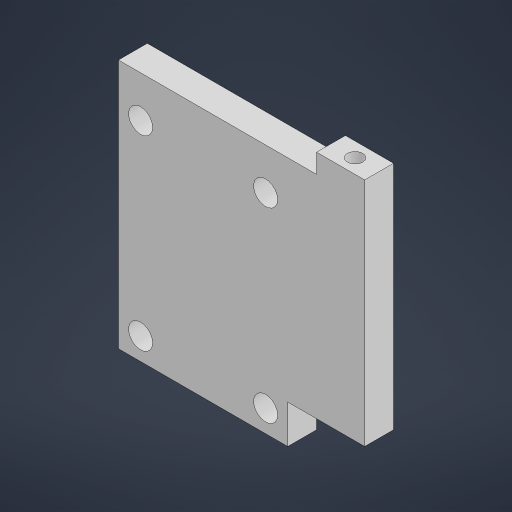
# Autodesk Inventor part: KickerMount_R
Saved by Autodesk Inventor 2024.2 (Build 282272000, 272)
## iProperties
Created: 2023-12-22
Part Number: KickerMount_R
Material: 一般
Document SubType Name: Modeling
Designer: Hanaoka
Density: 1 g/cm^3
Appearance: 既定
Author: Hanaoka
Autodesk Inventor part; units mm, degrees
ref_plane "YZ Plane" through (0, 0, 0) normal (1, 0, 0) x (0, 1, 0)
ref_plane "XZ Plane" through (0, 0, 0) normal (0, 1, 0) x (-1, 0, 0)
ref_plane "作業平面1" through (0, 0, 0) normal (0, 0, 1) x (1, 0, 0)
sketch "スケッチ1" plane through (0, 0, 0) normal (0, 0, 1) x (1, 0, 0)
  circle A0 centre (-6, -21.7) radius 1.25 projected
  circle A1 centre (-19, -21.7) radius 1.25 projected
  circle A2 centre (-19, -2.3) radius 1.25 projected
  circle A3 centre (-6, -2.3) radius 1.25 projected
  line L0 (0, -24) -> (-27.3, -24) projected
  line L1 (-3.7, -24) -> (-3.7, 2)
  line L2 (-3.7, 2) -> (-21.3, 2)
  line L3 (-21.3, 2) -> (-21.3, -24)
  circle A4 centre (-6, -21.7) radius 2.3 construction
  circle A5 centre (-19, -21.7) radius 2.3 construction
  line L4 (-3.7, -20) -> (4.3, -20)
  line L5 (4.3, -20) -> (4.3, 4)
  line L6 (4.3, 4) -> (-0.7, 4)
  line L7 (-0.7, 4) -> (-0.7, 2)
  line L8 (-0.7, 2) -> (-3.7, 2)
  point P0 (0, 0)
  dimension "d0" = 26
  dimension "d3" = 3
  dimension "d4" = 5
  dimension "d5" = 2
  dimension "d6" = 24
  constraints: 16 end point, 3 perpendicular, 3 point on line, 3 tangent, 2 centre point, 2 coincident, 2 horizontal, 2 vertical, 1 collinear, 1 equal radius
  measures "d0" distance of L1.start L1.end
  measures "d3" distance of L7.end L1.end
  measures "d4" distance of L5.end L6.end
  measures "d5" distance of L6.end L7.end
  measures "d6" distance of L4.end L5.end
extrude "押し出し1" add sketch "スケッチ1" along normal blind 3
sketch "スケッチ2" plane through (-0.7, 4, 0) normal (0, 1, 0) x (1, 0, 0)
  line L0 (5, 0) -> (0, 0) projected
  line L1 (0, 0) -> (0, -3) projected
  line L2 (5, -3) -> (0, -3) projected
  line L3 (5, 0) -> (5, -3) projected
  circle A0 centre (2.5, -1.5) radius 0.8
  line L4 (5, -3) -> (0, 0) construction
  line L5 (5, 0) -> (0, -3) construction
  point P0 (0.7, 0)
  dimension "d7" = 1.6
  constraints: 4 end point, 1 centre point, 1 coincident, 1 midpoint
  measures "d7" diameter of A0
extrude "押し出し2" cut sketch "スケッチ2" against normal blind 5 contours A0
